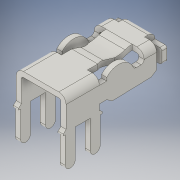
# Autodesk Inventor part: power claw
Saved by Autodesk Inventor 2019.3 (Build 233278000, 278)
## iProperties
Created: 2019-11-25
Part Number: power claw
Material: Generic
Document SubType Name: Modeling
Designer: kjdix
Density: 1 g/cm^3
Appearance: Steel
Author: kjdix
Autodesk Inventor part; units mm, degrees
ref_plane "YZ Plane" through (0, 0, 0) normal (1, 0, 0) x (0, 1, 0)
ref_plane "XZ Plane" through (0, 0, 0) normal (0, 1, 0) x (-1, 0, 0)
ref_plane "XY Plane" through (0, 0, 0) normal (0, 0, 1) x (1, 0, 0)
sketch "Sketch1" plane through (0, 0, 0) normal (1, 0, 0) x (0, 1, 0)
  line L0 (0, 3.048) -> (0, -3.048) construction
  line L1 (0, 4.2672) -> (-6.4008, 4.2672)
  line L2 (-7.62, 3.048) -> (-7.62, 3.048)
  line L3 (-6.4008, 1.8288) -> (0, 1.8288)
  line L4 (0, 1.8288) -> (0, 4.2672)
  line L5 (0, -1.8288) -> (-6.4008, -1.8288)
  line L6 (-7.62, -3.048) -> (-7.62, -3.048)
  line L7 (-6.4008, -4.2672) -> (0, -4.2672)
  line L8 (0, -4.2672) -> (0, -1.8288)
  arc A0 (-6.4008, 4.2672) -> (-7.62, 3.048) centre (-6.4008, 3.048) ccw
  arc A1 (-7.62, 3.048) -> (-6.4008, 1.8288) centre (-6.4008, 3.048) ccw
  arc A2 (-6.4008, -1.8288) -> (-7.62, -3.048) centre (-6.4008, -3.048) ccw
  arc A3 (-7.62, -3.048) -> (-6.4008, -4.2672) centre (-6.4008, -3.048) ccw
  line L9 (1.101, 4.064) -> (8.128, 4.064)
  line L10 (0, 1.8288) -> (0.5077, 1.8288)
  line L11 (0.5077, 1.8288) -> (0.5077, -1.8288)
  line L12 (0.5077, -1.8288) -> (0, -1.8288)
  line L13 (1.101, -4.064) -> (8.128, -4.064)
  line L14 (8.128, 4.064) -> (8.128, -4.064)
  line L15 (9.6945, 6.0164) -> (9.6945, -21.4972) construction
  line L16 (9.6945, -21.4972) -> (-9.2094, -21.4972) construction
  line L17 (-9.2094, -21.4972) -> (-9.2094, 6.0164) construction
  line L18 (-9.2094, 6.0164) -> (9.6945, 6.0164) construction
  line L19 (6.477, -20.574) -> (3.0558, -20.574)
  line L20 (0, 4.2672) -> (0, 4.572)
  line L21 (0, 4.2672) -> (0, 5.1984)
  line L22 (0.4363, 4.7489) -> (1.101, 4.064)
  arc A4 (0.4363, 4.7489) -> (0, 4.572) centre (0.254, 4.572) ccw
  line L23 (0.9401, 4.826) -> (-0.3391, 4.826) construction
  line L24 (0, -4.2672) -> (0, -4.572)
  line L25 (1.101, -4.064) -> (0.4363, -4.7489)
  arc A5 (0, -4.572) -> (0.4363, -4.7489) centre (0.254, -4.572) ccw
  line L26 (0.7296, -4.826) -> (-0.2296, -4.826) construction
  line L27 (2.413, -4.064) -> (2.413, -5.8788)
  line L28 (2.413, -5.8788) -> (1.4758, -7.2025)
  line L29 (1.4758, -7.2025) -> (1.7607, -16.7836)
  line L30 (1.7607, -16.7836) -> (2.617, -18.0539)
  line L31 (2.617, -18.0539) -> (8.128, -18.0539)
  line L32 (8.128, -18.0539) -> (8.128, -15.0059)
  line L33 (8.128, -15.0059) -> (6.35, -15.0059)
  line L34 (6.35, -4.064) -> (6.35, -5.8649)
  line L35 (6.35, -5.8649) -> (7.1177, -5.8649)
  line L36 (5.6054, -13.0152) -> (5.6054, -14.2613)
  arc A6 (5.6054, -14.2613) -> (6.35, -15.0059) centre (6.35, -14.2613) ccw
  arc A7 (6.0714, -12.3147) -> (7.1177, -5.8649) centre (4.5832, -8.7635) ccw
  arc A8 (6.0714, -12.3147) -> (5.6054, -13.0152) centre (6.365, -13.0152) ccw
  line L37 (6.35, -4.064) -> (2.413, -4.064)
  line L38 (6.477, -20.574) -> (3.048, -20.574)
  line L39 (3.048, -20.574) -> (3.048, -19.304)
  line L40 (3.048, -19.304) -> (6.477, -19.304)
  line L41 (6.477, -19.304) -> (6.477, -20.574)
  line L42 (8.128, 4.064) -> (6.858, 4.064)
  line L43 (6.858, 4.064) -> (6.858, -4.064)
  line L44 (6.858, -4.064) -> (8.128, -4.064)
  line L45 (8.128, -4.064) -> (8.128, 4.064)
  line L46 (8.128, -15.0059) -> (6.858, -15.0059)
  line L47 (6.858, -15.0059) -> (6.858, -18.0539)
  line L48 (6.858, -18.0539) -> (8.128, -18.0539)
  line L49 (8.128, -18.0539) -> (8.128, -15.0059)
  point P0 (0, 0)
  point P1 (0, 0)
  point P2 (-7.62, 1.8288)
  point P3 (-7.62, 4.2672)
  point P4 (-7.62, -4.2672)
  point P5 (-7.62, -1.8288)
  point P6 (0.3427, 4.445)
  point P7 (0.3427, -4.445)
  dimension "d0" = 6.096
  dimension "d1" = 7.62
  dimension "d2" = 2.4384
  dimension "d3" = 7.62
  dimension "d4" = 2.4384
  dimension "d5" = 1.2192
  dimension "d53" = 24.638
  dimension "d85" = 8.128
  dimension "d89" = 0.2032
  dimension "d90" = 0.2032
  dimension "d91" = 0.254
  dimension "d93" = 0.5588
  dimension "d97" = 0.254
  dimension "d98" = 0.5588
  dimension "d117" = 1.27
  dimension "d118" = 3.429
  dimension "d119" = 3.937
  dimension "d120" = 3.048
  dimension "d123" = 1.27
  dimension "d128" = 1.27
  dimension "d131" = 0.508
  dimension "d132" = 0.508
  dimension "d138" = 0.381
  constraints: 92 end point, 18 point on circle, 18 tangent, 14 point on line, 12 perpendicular, 10 parallel, 9 centre point, 9 horizontal, 8 vertical, 3 equal radius, 3 midpoint, 1 coincident, 1 collinear, 1 equal length, 2 other
  measures "d0" distance of L0.end L0.start
  measures "d1" distance of L3.end point (-7.62, 1.829)
  measures "d2" distance of point (-7.62, 1.829) point (-7.62, 4.267)
  measures "d3" distance of L7.end point (-7.62, -4.267)
  measures "d4" distance of point (-7.62, -4.267) point (-7.62, -1.829)
  measures "d5" radius of A0
  measures "d53" distance between parallel lines of L19 L9
  measures "d85" distance between parallel lines of L14 L4
  measures "d89" distance from line of L9 L1.start
  measures "d90" distance between parallel lines of L13 L7
  measures "d91" radius of A4
  measures "d93" distance between parallel lines of L1 L23
  measures "d97" radius of A5
  measures "d98" distance between parallel lines of L7 L26
  measures "d117" distance of L40.end L19.start
  measures "d118" distance of L39.end L40.end
  measures "d119" distance between parallel lines of L27 L34
  measures "d120" distance of L31.end L32.end
  measures "d123" distance of L44.end L43.end
  measures "d128" distance of L48.end L47.end
  measures "d131" distance between parallel lines of L43 L34
  measures "d132" distance from line of L47 L33.end
  measures "d138" distance between parallel lines of L41 L47
extrude "Extrusion1" add sketch "Sketch1" along normal mid plane 12.192 contours L4 L3 A1 A0 L1 | L20 A4 L22 L9 L43 L13 L25 A5 L24 L8 L12 L11 L10 L4 | L8 L7 A3 A2 L5 | L9 L14 L13 L43 | L34 L35 A7 A8 L36 A6 L33 L47 L31 L30 L29 L28 L27 L13 | L47 L33 L32 L31
extrude "Extrusion2" cut sketch "Sketch1" along normal mid plane 9.652 contours L4 L3 A1 A0 L1 | L20 A4 L22 L9 L43 L13 L25 A5 L24 L8 L12 L11 L10 L4 | L8 L7 A3 A2 L5 | L9 L14 L13 L43 | L34 L35 A7 A8 L36 A6 L33 L47 L31 L30 L29 L28 L27 L13 | L47 L33 L32 L31
extrude "Extrusion3" add sketch "Sketch1" along normal mid plane 12.192 contours L9 L14 L13 L43 | L47 L33 L32 L31 | L19 L38 L39 L40 L41
fillet "Fillet1" radius 0.508 4 edges at (4.826, 6.858, 0) (-4.826, 6.858, 0) (-4.826, 6.858, -16.5299) (4.826, 6.858, -16.5299)
fillet "Fillet2" radius 1.778 2 edges at (6.096, 8.128, 0) (-6.096, 8.128, 0)
fillet "Fillet3" radius 1.778 2 edges at (6.096, 8.128, -16.5299) (-6.096, 8.128, -16.5299)
fillet "Fillet4" radius 0.508 4 edges at (6.096, 6.477, -19.939) (-6.096, 6.477, -19.939) (6.096, 3.048, -19.939) (-6.096, 3.048, -19.939)
sketch "Sketch2" plane through (0, 0, 0) normal (1, 0, 0) x (0, 1, 0)
  line L0 (6.477, -19.304) -> (6.477, -20.574) projected
  arc A0 (6.477, -19.939) -> (7.493, -18.923) centre (6.477, -18.923) ccw
  line L1 (7.493, -18.923) -> (7.493, -18.0539)
  line L2 (8.128, -18.0539) -> (6.35, -18.0539) projected
  line L3 (8.128, -18.0539) -> (6.858, -18.0539) projected
  line L4 (6.858, -18.0539) -> (6.858, -15.0059) projected
  line L5 (6.858, -15.0059) -> (8.128, -15.0059) projected
  line L6 (8.128, -15.0059) -> (8.128, -18.0539) projected
  line L7 (8.128, -4.064) -> (6.858, -4.064) projected
  line L8 (6.858, -4.064) -> (6.858, 4.064) projected
  line L9 (6.858, 4.064) -> (8.128, 4.064) projected
  line L10 (8.128, 4.064) -> (8.128, -4.064) projected
  line L11 (3.048, -19.304) -> (6.477, -19.304) projected
  line L12 (6.477, -19.304) -> (6.477, -20.574) projected
  line L13 (6.477, -20.574) -> (3.048, -20.574) projected
  line L14 (3.048, -20.574) -> (3.048, -19.304) projected
  line L15 (7.493, -18.0539) -> (7.493, -15.0059)
  line L16 (8.128, -4.064) -> (6.35, -4.064) projected
  line L17 (7.493, -4.064) -> (7.493, -6.604)
  arc A1 (7.2207, -8.138) -> (7.493, -6.604) centre (3.036, -6.604) ccw
  arc A2 (7.2207, -8.138) -> (7.2207, -13.4719) centre (14.4962, -10.8049) ccw
  arc A3 (7.493, -15.0059) -> (7.2207, -13.4719) centre (3.036, -15.0059) ccw
  point P0 (0, 0)
  dimension "d139" = 1.016
  dimension "d140" = 2.54
  constraints: 8 point on circle, 6 end point, 5 tangent, 4 centre point, 3 midpoint, 2 point on line, 2 vertical, 1 equal radius, 1 line through centre
  measures "d139" radius of A0
  measures "d140" distance of L17.start L17.end
sketch "Sketch3" plane through (4.318, 6.858, -4.064) normal (0, 0, -1) x (-1, 0, 0)
  line L0 (1.143, 0) -> (7.493, 0)
  line L1 (7.493, 0) -> (7.493, 1.27)
  line L2 (7.493, 1.27) -> (1.143, 1.27)
  line L3 (1.143, 1.27) -> (1.143, 0)
  line L4 (1.143, 0) -> (7.493, 1.27) construction
  line L5 (7.493, 0) -> (1.143, 1.27) construction
  point P0 (4.318, -6.858)
  point P1 (4.318, 0.635)
  dimension "d141" = 6.35
  dimension "d142" = 1.27
  constraints: 12 end point, 2 midpoint, 2 parallel, 1 horizontal, 1 perpendicular
  measures "d141" distance of L2.end L1.end
  measures "d142" distance of L1.end L0.end
sweep "Sweep1" add profiles "Sketch3" path "Sketch2" path curves L17 A1 A2 A3 L15 L1 A0
sketch "Sketch4" plane through (-4.318, 8.128, 4.064) normal (0, 1, 0) x (1, 0, 0)
  line L0 (1.143, 11.9834) -> (1.143, 10.668) projected
  line L1 (1.143, 12.4205) -> (1.143, 17.3174) projected
  arc A0 (1.143, 10.668) -> (1.143, 14.8689) centre (-3.4824, 12.7685) ccw
  line L2 (7.493, 12.4205) -> (7.493, 17.3174) projected
  line L3 (7.493, 12.4205) -> (7.493, 10.668) projected
  arc A1 (7.493, 14.8689) -> (7.493, 10.668) centre (12.1184, 12.7685) ccw
  line L4 (1.143, 10.668) -> (7.493, 10.668) projected
  arc A2 (7.493, 10.668) -> (7.493, 14.8689) centre (4.3638, 12.7685) ccw
  arc A3 (1.143, 14.8689) -> (1.143, 10.668) centre (4.153, 12.7685) ccw
  point P0 (4.318, 4.064)
  dimension "d145" = 5.08
  dimension "d146" = 5.08
  constraints: 8 point on circle, 4 centre point, 3 midpoint
  measures "d145" radius of A0
  measures "d146" radius of A1
extrude "Extrusion4" cut sketch "Sketch4" against normal through all contours A3 A0 | L3 A1 L2
body "Solid1"
